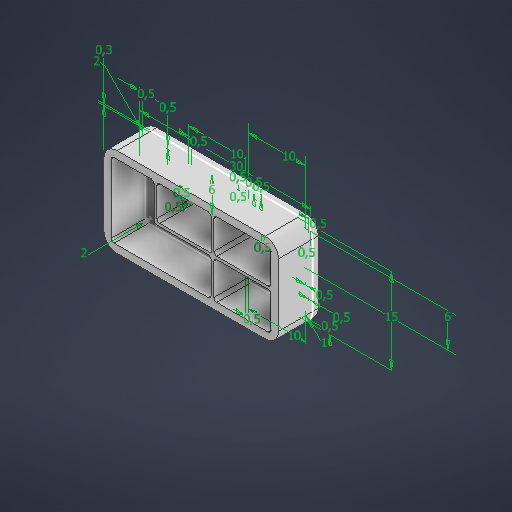
# Autodesk Inventor part: prototipo
Saved by Autodesk Inventor 2026.2 (Build 302298010, 298A)
## iProperties
Created: 2026-03-13
Part Number: prototipo
Material: Genérico
Document SubType Name: Modeling
Designer: Lucas David
Density: 1 g/cm^3
Appearance: Padrão
Author: Lucas David
Autodesk Inventor part; units mm, degrees
ref_plane "YZ Plane" through (0, 0, 0) normal (1, 0, 0) x (0, 1, 0)
ref_plane "XZ Plane" through (0, 0, 0) normal (0, 1, 0) x (-1, 0, 0)
ref_plane "XY Plane" through (0, 0, 0) normal (0, 0, 1) x (1, 0, 0)
sketch "Esboço4" plane through (0, 0, 0) normal (0, 0, 1) x (1, 0, 0)
  line L0 (-130, -75) -> (130, -75)
  line L1 (150, -55) -> (150, 55)
  line L2 (130, 75) -> (-130, 75)
  line L3 (-150, 55) -> (-150, -55)
  line L4 (-150, -75) -> (150, 75) construction
  line L5 (150, -75) -> (-150, 75) construction
  arc A0 (-130, 75) -> (-150, 55) centre (-130, 55) ccw
  arc A1 (-150, -55) -> (-130, -75) centre (-130, -55) ccw
  arc A2 (130, -75) -> (150, -55) centre (130, -55) ccw
  arc A3 (150, 55) -> (130, 75) centre (130, 55) ccw
  line L6 (-153, -55) -> (-153, 55)
  arc A4 (-130, 78) -> (-153, 55) centre (-130, 55) ccw
  line L7 (-130, 78) -> (130, 78)
  arc A5 (153, 55) -> (130, 78) centre (130, 55) ccw
  line L8 (153, 55) -> (153, -55)
  arc A6 (130, -78) -> (153, -55) centre (130, -55) ccw
  line L9 (130, -78) -> (-130, -78)
  arc A7 (-153, -55) -> (-130, -78) centre (-130, -55) ccw
  line L10 (45, 65) -> (135, 65)
  line L11 (140, 60) -> (140, 10)
  line L12 (135, 5) -> (45, 5)
  line L13 (40, 10) -> (40, 60)
  line L14 (135, 70) -> (35, 70)
  line L15 (35, 60) -> (35, 5)
  line L16 (45, 0) -> (135, 0)
  line L17 (145, -5) -> (145, 60)
  line L18 (40, 0) -> (140, 0)
  line L19 (145, -5) -> (145, -60)
  line L20 (135, -70) -> (30, -70)
  line L21 (35, -60) -> (35, -5)
  line L22 (140, -5) -> (140, -60)
  line L23 (135, -65) -> (45, -65)
  line L24 (40, -60) -> (40, -5)
  line L25 (35, 70) -> (-70, 70)
  line L26 (-65, 60) -> (-65, 5)
  line L27 (-60, 0) -> (30, 0)
  line L28 (35, 5) -> (-55, 5)
  line L29 (-60, 10) -> (-60, 60)
  line L30 (-55, 65) -> (30, 65)
  line L31 (30, -70) -> (-135, -70)
  line L32 (-145, -60) -> (-145, 60)
  line L33 (-135, 70) -> (-70, 70)
  line L34 (-70, 65) -> (-135, 65)
  line L35 (-140, 60) -> (-140, -60)
  line L36 (-135, -65) -> (30, -65)
  arc A8 (135, -70) -> (145, -60) centre (135, -60) ccw
  arc A9 (145, 60) -> (135, 70) centre (135, 60) ccw
  arc A10 (-135, 70) -> (-145, 60) centre (-135, 60) ccw
  arc A11 (-145, -60) -> (-135, -70) centre (-135, -60) ccw
  arc A12 (-65, 5) -> (-60, 0) centre (-60, 5) ccw
  arc A13 (-60, 10) -> (-55, 5) centre (-55, 10) ccw
  arc A14 (40, 10) -> (45, 5) centre (45, 10) ccw
  arc A15 (35, -5) -> (30, 0) centre (30, -5) ccw
  arc A16 (45, 0) -> (40, -5) centre (45, -5) ccw
  arc A17 (35, 60) -> (30, 65) centre (30, 60) ccw
  arc A18 (45, 65) -> (40, 60) centre (45, 60) ccw
  arc A19 (-55, 65) -> (-60, 60) centre (-55, 60) ccw
  arc A20 (-65, 60) -> (-70, 65) centre (-70, 60) ccw
  arc A21 (140, 60) -> (135, 65) centre (135, 60) ccw
  arc A22 (135, 5) -> (140, 10) centre (135, 10) ccw
  arc A23 (140, -5) -> (135, 0) centre (135, -5) ccw
  arc A24 (135, -65) -> (140, -60) centre (135, -60) ccw
  arc A25 (40, -60) -> (45, -65) centre (45, -60) ccw
  arc A26 (30, -65) -> (35, -60) centre (30, -60) ccw
  arc A27 (-140, -60) -> (-135, -65) centre (-135, -60) ccw
  arc A28 (-135, 65) -> (-140, 60) centre (-135, 60) ccw
  point P0 (0, 0)
  point P1 (40, 65)
  point P2 (140, 5)
  point P3 (140, 65)
  point P4 (40, 5)
  point P5 (35, 0)
  point P6 (140, -65)
  point P7 (40, -65)
  point P8 (-65, 0)
  point P9 (-60, 5)
  point P10 (-60, 65)
  point P11 (-140, 65)
  point P12 (-140, -65)
  point P13 (35, 65)
  point P14 (35, -65)
  point P15 (-65, 65)
  point P16 (35, -11.1171)
  dimension "d13" = 150
  dimension "d14" = 300
  dimension "d17" = 20
  dimension "d18" = 20
  dimension "d19" = 3
  dimension "d20" = 60
  dimension "d21" = 100
  dimension "d25" = 5
  dimension "d26" = 5
  dimension "d27" = 5
  dimension "d28" = 5
  dimension "d31" = 5
  dimension "d32" = 5
  dimension "d33" = 5
  dimension "d38" = 100
  dimension "d39" = 5
  dimension "d41" = 5
  dimension "d42" = 5
  dimension "d43" = 5
  dimension "d44" = 5
  dimension "d47" = 5
  dimension "d49" = 100
  dimension "d50" = 5
  dimension "d57" = 10
  dimension "d62" = 60
  dimension "d63" = 5
  dimension "d64" = 5
  constraints: 74 end point, 58 point on circle, 50 tangent, 42 point on line, 29 centre point, 21 equal radius, 13 parallel, 9 perpendicular, 5 horizontal, 2 midpoint, 1 vertical, 10 other
  measures "d13" distance between parallel lines of L0 L2
  measures "d14" distance between parallel lines of L1 L3
  measures "d17" radius of A0
  measures "d18" radius of A1
  measures "d19" distance between parallel lines of L2 L7
  measures "d20" distance between parallel lines of L12 L10
  measures "d21" distance between parallel lines of L11 L13
  measures "d25" distance between parallel lines of L2 L14
  measures "d26" distance between parallel lines of L11 L17
  measures "d27" distance between parallel lines of L1 L17
  measures "d28" distance between parallel lines of L0 L20
  measures "d31" distance between parallel lines of L19 L22
  measures "d32" distance between parallel lines of L1 L19
  measures "d33" distance between parallel lines of L12 L16
  measures "d38" distance between parallel lines of L15 L26
  measures "d39" distance between parallel lines of L26 L29
  measures "d41" distance between parallel lines of L3 L32
  measures "d42" distance between parallel lines of L33 L34
  measures "d43" distance between parallel lines of L13 L15
  measures "d44" distance between parallel lines of L14 L10
  measures "d47" distance between parallel lines of L25 L30
  measures "d49" distance between parallel lines of L22 L24
  measures "d50" distance between parallel lines of L24 L21
  measures "d57" radius of A8
  measures "d62" distance between parallel lines of L30 L28
  measures "d63" distance between parallel lines of L28 L27
  measures "d64" radius of A12
extrude "Extrusão4" add sketch "Esboço4" along normal blind 60 contours A1 L3 A0 L2 A3 L1 A2 L0 | L6 A4 L7 A5 L8 A6 L9 A7 | L10 A21 L11 A22 L12 A14 L13 A18 | A9 L17 L19 A8 L20 L31 A11 L32 A10 L33 L25 L14 | L15 L28 A13 L29 A19 L30 A17 | L16 A23 L22 A24 L23 A25 L24 A16 | A26 L36 A27 L35 A28 L34 A20 L26 A12 L27 A15 L21
extrude "Extrusão5" cut sketch "Esboço4" along normal blind 80 contours L10 A21 L11 A22 L12 A14 L13 A18 | L15 L28 A13 L29 A19 L30 A17 | L16 A23 L22 A24 L23 A25 L24 A16 | A26 L36 A27 L35 A28 L34 A20 L26 A12 L27 A15 L21
extrude "Extrusão6" add sketch "Esboço4" against normal blind 10 contours A1 L3 A0 L2 A3 L1 A2 L0 | L6 A4 L7 A5 L8 A6 L9 A7 | L10 A21 L11 A22 L12 A14 L13 A18 | A9 L17 L19 A8 L20 L31 A11 L32 A10 L33 L25 L14 | L15 L28 A13 L29 A19 L30 A17 | L16 A23 L22 A24 L23 A25 L24 A16 | A26 L36 A27 L35 A28 L34 A20 L26 A12 L27 A15 L21
sketch "Esboço1" plane through (0, 0, 0) normal (0, 0, 1) x (1, 0, 0)
  line L0 (-25, -12.5) -> (25, -12.5)
  line L1 (25, -12.5) -> (25, 12.5)
  line L2 (25, 12.5) -> (-25, 12.5)
  line L3 (-25, 12.5) -> (-25, -12.5)
  line L4 (-25, -12.5) -> (25, 12.5) construction
  line L5 (25, -12.5) -> (-25, 12.5) construction
  point P0 (0, 0)
  dimension "d0" = 25
  dimension "d1" = 50
  constraints: 12 end point, 2 midpoint, 2 parallel, 1 horizontal, 1 perpendicular
  measures "d0" distance between parallel lines of L0 L2
  measures "d1" distance between parallel lines of L3 L1
sketch "Esboço2" plane through (0, 0, 100) normal (0, 0, 1) x (1, 0, 0)
  line L0 (25, -12.5) -> (25, 12.5) projected
  line L1 (25, 12.5) -> (-25, 12.5) projected
  line L2 (-25, 12.5) -> (-25, -12.5) projected
  line L3 (-25, -12.5) -> (25, -12.5) projected
  line L4 (-27, 14.5) -> (27, 14.5)
  line L5 (27, 14.5) -> (27, -14.5)
  line L6 (27, -14.5) -> (-27, -14.5)
  line L7 (-27, -14.5) -> (-27, 14.5)
  point P0 (0, 0)
  dimension "d4" = 2
  constraints: 8 end point, 3 other
  measures "d4" distance between parallel lines of L1 L4
